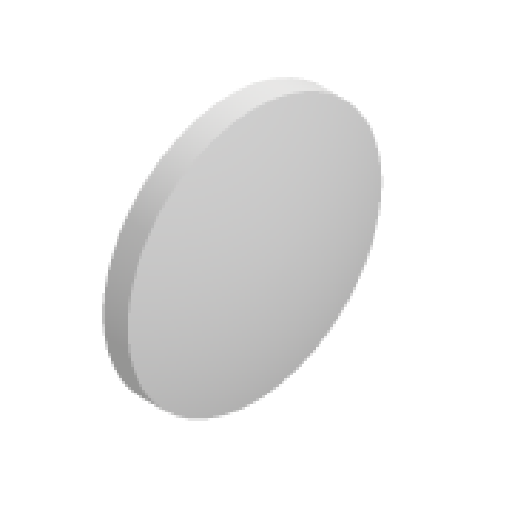
# Autodesk Inventor part: 00_Lens_f25_d15mm
Saved by Autodesk Inventor 2025.1 (Build 291241020, 241B)
## iProperties
Created: 2024-10-03
Part Number: 00_Lens_f25_d15mm
Material: Generic
Document SubType Name: Modeling
Designer: diederichbenedict
Density: 1 g/cm^3
Appearance: Default
Author: diederichbenedict
Autodesk Inventor part; units mm, degrees
ref_plane "YZ Plane" through (0, 0, 0) normal (1, 0, 0) x (0, 1, 0)
ref_plane "XZ Plane" through (0, 0, 0) normal (0, 1, 0) x (-1, 0, 0)
ref_plane "XY Plane" through (0, 0, 0) normal (0, 0, 1) x (1, 0, 0)
sketch "Sketch1" plane through (0, 0, 0) normal (0, 0, 1) x (1, 0, 0)
  arc A0 (0, 0) -> (-1.5751, 7.5) centre (-19.4723, -0.1741) ccw
  line L0 (-1.5751, 7.5) -> (-3, 7.5)
  line L1 (0, 0) -> (0, 0)
  line L2 (-3, 7.5) -> (-3, 0)
  line L3 (-3, 0) -> (0, 0)
  line L4 (-23.4413, 0) -> (4.3416, 0) projected
  point P0 (-1.5, 0)
  dimension "d0" = 7.5
  dimension "d1" = 3
  constraints: 8 end point, 2 point on circle, 1 centre point, 1 horizontal, 1 midpoint, 1 perpendicular, 1 vertical
  measures "d0" distance from line of point (-1.5, 0) L0
  measures "d1" distance from line of L1.start L2
revolve "Revolution1" add sketch "Sketch1" angle 360 about axis through (-10, 0, 0) along (1, 0, 0)
body "Solid1"
